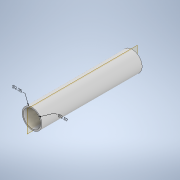
# Autodesk Inventor part: 2inchPvcForBracket
Saved by Autodesk Inventor 2022.2 (Build 262287000, 287)
## iProperties
Created: 2021-11-22
Part Number: 2inchPvcForBracket
Material: Generic
Document SubType Name: Modeling
Designer: robst
Density: 1 g/cm^3
Appearance: Default
Author: robst
Autodesk Inventor part; units mm, degrees
ref_plane "XZ Plane" through (0, 0, 0) normal (0, 1, 0) x (-1, 0, 0)
ref_plane "XY Plane" through (0, 0, 0) normal (0, 0, 1) x (1, 0, 0)
sketch "Sketch1" plane through (0, 0, 0) normal (0, 0, 1) x (1, 0, 0)
  circle A0 centre (0, 0) radius 30.2895
  circle A1 centre (0, 0) radius 26.2509
  dimension "d0" = 60.579
  dimension "d1" = 52.5018
  constraints: 2 centre point, 2 coincident
  measures "d0" diameter of A0
  measures "d1" diameter of A1
extrude "Extrusion1" add sketch "Sketch1" along normal mid plane 304.8
equation "\"d0\" = pipeOutsideDiameter"
equation "\"d1\" = pipeInsideDiameter"
equation "\"pipeOutsideDiameter\" = 60.579"
equation "\"pipeInsideDiameter\" = 52.5018"
body "Solid1"
